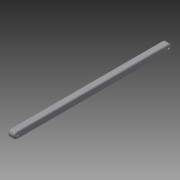
# Autodesk Inventor part: bar
Saved by Autodesk Inventor 2015 (Build 190159000, 159)
## iProperties
Created: 2015-04-08
Part Number: bar
Material: Generic
Document SubType Name: Modeling
Designer: WASHHSST
Density: 1 g/cm^3
Appearance: Default
Mass: 380.146 g
Surface Area: 595.505 cm^2
Volume: 380.146 cm^3
Author: WASHHSST
Autodesk Inventor part; units mm, degrees
ref_plane "YZ Plane" through (0, 0, 0) normal (1, 0, 0) x (0, 1, 0)
ref_plane "XZ Plane" through (0, 0, 0) normal (0, 1, 0) x (-1, 0, 0)
sketch "Sketch1" plane through (0, 0, 0) normal (1, 0, 0) x (0, 1, 0)
  line L0 (0, 0) -> (25.4, 0)
  line L1 (25.4, 0) -> (25.4, -609.6)
  line L2 (25.4, -609.6) -> (0, -609.6)
  line L3 (0, -609.6) -> (0, 0)
  dimension "d0" = 25.4
  dimension "d1" = 609.6
  constraints: 8 end point, 2 parallel, 1 horizontal, 1 perpendicular
  measures "d0" distance of L1.end L2.end
  measures "d1" distance of L0.end L1.end
extrude "Extrusion1" add sketch "Sketch1" along normal blind 25.4
sketch "Sketch3" plane through (25.4, 0, 0) normal (1, 0, 0) x (0, 0, -1)
  circle A0 centre (12.7, 12.7) radius 12.7
  line L0 (609.6, 25.4) -> (0, 25.4) projected
  line L1 (0, 25.4) -> (0, 0) projected
  circle A1 centre (12.7, 12.7) radius 3.175
  dimension "d12" = 25.4
  dimension "d13" = 6.35
  constraints: 2 centre point, 2 tangent, 1 concentric
  measures "d12" diameter of A0
  measures "d13" diameter of A1
extrude "Extrusion3" cut sketch "Sketch3" against normal blind 25.4 contours A1
ref_plane "Work Plane1" through (0, 0, -304.8) normal (0, 0, 1) x (1, 0, 0)
mirror "Mirror1" about plane through (0, 0, -304.8) normal (0, 0, 1) of "Extrusion3"
fillet "Fillet1" radius 12.7 4 edges at (12.7, 25.4, 0) (12.7, 0, 0) (12.7, 25.4, -609.6) (12.7, 0, -609.6)
chamfer "Chamfer1" distance 2.54 angle 45 8 edges at (25.4, 25.4, -304.8) (25.4, 21.6803, -3.7197) (25.4, 0, -304.8) (25.4, 21.6803, -605.8803) (0, 25.4, -304.8) (0, 21.6803, -605.8803) (0, 0, -304.8) (0, 21.6803, -3.7197)
body "Solid1"
